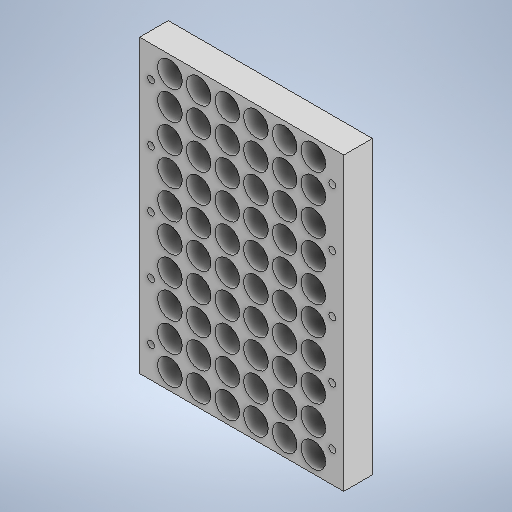
# Autodesk Inventor part: Battery Holder pt1
Saved by Autodesk Inventor 2025.2 (Build 292293000, 293)
## iProperties
Created: 2025-03-23
Part Number: Battery Holder pt1
Material: Generic
Document SubType Name: Modeling
Designer: Mathias
Density: 1 g/cm^3
Appearance: Default
Author: Mathias
Autodesk Inventor part; units mm, degrees
ref_plane "YZ Plane" through (0, 0, 0) normal (1, 0, 0) x (0, 1, 0)
ref_plane "XZ Plane" through (0, 0, 0) normal (0, 1, 0) x (-1, 0, 0)
ref_plane "XY Plane" through (0, 0, 0) normal (0, 0, 1) x (1, 0, 0)
sketch "Sketch1" plane through (0, 0, 0) normal (0, 0, 1) x (1, 0, 0)
  line L0 (0, 0) -> (178, 0)
  line L1 (178, 0) -> (178, 254)
  line L2 (178, 254) -> (0, 254)
  line L3 (0, 254) -> (0, 0)
  circle A0 centre (26.5, 14.5) radius 10.7
  circle A1 centre (26.5, 39.5) radius 10.7
  circle A2 centre (26.5, 64.5) radius 10.7
  circle A3 centre (26.5, 89.5) radius 10.7
  circle A4 centre (26.5, 114.5) radius 10.7
  circle A5 centre (26.5, 139.5) radius 10.7
  circle A6 centre (26.5, 164.5) radius 10.7
  circle A7 centre (26.5, 189.5) radius 10.7
  circle A8 centre (26.5, 214.5) radius 10.7
  circle A9 centre (26.5, 239.5) radius 10.7
  circle A10 centre (51.5, 14.5) radius 10.7
  circle A11 centre (51.5, 39.5) radius 10.7
  circle A12 centre (51.5, 64.5) radius 10.7
  circle A13 centre (51.5, 89.5) radius 10.7
  circle A14 centre (51.5, 114.5) radius 10.7
  circle A15 centre (51.5, 139.5) radius 10.7
  circle A16 centre (51.5, 164.5) radius 10.7
  circle A17 centre (51.5, 189.5) radius 10.7
  circle A18 centre (51.5, 214.5) radius 10.7
  circle A19 centre (51.5, 239.5) radius 10.7
  circle A20 centre (76.5, 14.5) radius 10.7
  circle A21 centre (76.5, 39.5) radius 10.7
  circle A22 centre (76.5, 64.5) radius 10.7
  circle A23 centre (76.5, 89.5) radius 10.7
  circle A24 centre (76.5, 114.5) radius 10.7
  circle A25 centre (76.5, 139.5) radius 10.7
  circle A26 centre (76.5, 164.5) radius 10.7
  circle A27 centre (76.5, 189.5) radius 10.7
  circle A28 centre (76.5, 214.5) radius 10.7
  circle A29 centre (76.5, 239.5) radius 10.7
  circle A30 centre (101.5, 14.5) radius 10.7
  circle A31 centre (101.5, 39.5) radius 10.7
  circle A32 centre (101.5, 64.5) radius 10.7
  circle A33 centre (101.5, 89.5) radius 10.7
  circle A34 centre (101.5, 114.5) radius 10.7
  circle A35 centre (101.5, 139.5) radius 10.7
  circle A36 centre (101.5, 164.5) radius 10.7
  circle A37 centre (101.5, 189.5) radius 10.7
  circle A38 centre (101.5, 214.5) radius 10.7
  circle A39 centre (101.5, 239.5) radius 10.7
  circle A40 centre (126.5, 14.5) radius 10.7
  circle A41 centre (126.5, 39.5) radius 10.7
  circle A42 centre (126.5, 64.5) radius 10.7
  circle A43 centre (126.5, 89.5) radius 10.7
  circle A44 centre (126.5, 114.5) radius 10.7
  circle A45 centre (126.5, 139.5) radius 10.7
  circle A46 centre (126.5, 164.5) radius 10.7
  circle A47 centre (126.5, 189.5) radius 10.7
  circle A48 centre (126.5, 214.5) radius 10.7
  circle A49 centre (126.5, 239.5) radius 10.7
  circle A50 centre (151.5, 14.5) radius 10.7
  circle A51 centre (151.5, 39.5) radius 10.7
  circle A52 centre (151.5, 64.5) radius 10.7
  circle A53 centre (151.5, 89.5) radius 10.7
  circle A54 centre (151.5, 114.5) radius 10.7
  circle A55 centre (151.5, 139.5) radius 10.7
  circle A56 centre (151.5, 164.5) radius 10.7
  circle A57 centre (151.5, 189.5) radius 10.7
  circle A58 centre (151.5, 214.5) radius 10.7
  circle A59 centre (151.5, 239.5) radius 10.7
  circle A60 centre (10, 27) radius 3
  circle A61 centre (10, 77) radius 3
  circle A62 centre (10, 127) radius 3
  circle A63 centre (10, 177) radius 3
  circle A64 centre (10, 227) radius 3
  circle A65 centre (168, 27) radius 3
  circle A66 centre (168, 77) radius 3
  circle A67 centre (168, 127) radius 3
  circle A68 centre (168, 177) radius 3
  circle A69 centre (168, 227) radius 3
  dimension "d0" = 178
  dimension "d1" = 254
  dimension "d2" = 21.4
  dimension "d5" = 25
  dimension "d8" = 25
  dimension "d31" = 6
  dimension "d34" = 50
  dimension "d37" = 158
  constraints: 70 centre point, 8 end point, 3 horizontal, 3 perpendicular, 2 vertical, 136 other
  measures "d0" distance of L0.start L0.end
  measures "d1" distance of L0.end L1.end
  measures "d2" diameter of A0
  measures "d5" distance of A0.centre A1.centre
  measures "d8" distance of A0.centre A10.centre
  measures "d31" diameter of A60
  measures "d34" distance of A60.centre A61.centre
  measures "d37" distance of A60.centre A65.centre
extrude "Extrusion1" add sketch "Sketch1" along normal blind 20
sketch "Sketch2" plane through (0, 0, 0) normal (0, 0, -1) x (-1, 0, 0)
  line L0 (-178, 0) -> (-178, 254) projected
  line L1 (-178, 254) -> (0, 254)
  line L2 (0, 254) -> (0, 0)
  line L3 (0, 0) -> (-178, 0)
  line L4 (-178, 0) -> (-178, 254)
  line L5 (-161, 5) -> (-92, 5)
  line L6 (-92, 5) -> (-92, 49)
  line L7 (-92, 49) -> (-161, 49)
  line L8 (-161, 49) -> (-161, 5)
  line L9 (-161, 99) -> (-161, 55)
  line L10 (-92, 99) -> (-161, 99)
  line L11 (-92, 55) -> (-92, 99)
  line L12 (-161, 55) -> (-92, 55)
  line L13 (-161, 149) -> (-161, 105)
  line L14 (-92, 149) -> (-161, 149)
  line L15 (-92, 105) -> (-92, 149)
  line L16 (-161, 105) -> (-92, 105)
  line L17 (-161, 199) -> (-161, 155)
  line L18 (-92, 199) -> (-161, 199)
  line L19 (-92, 155) -> (-92, 199)
  line L20 (-161, 155) -> (-92, 155)
  line L21 (-161, 249) -> (-161, 205)
  line L22 (-92, 249) -> (-161, 249)
  line L23 (-92, 205) -> (-92, 249)
  line L24 (-161, 205) -> (-92, 205)
  line L25 (-86, 49) -> (-86, 5)
  line L26 (-17, 49) -> (-86, 49)
  line L27 (-17, 5) -> (-17, 49)
  line L28 (-86, 5) -> (-17, 5)
  line L29 (-86, 99) -> (-86, 55)
  line L30 (-17, 99) -> (-86, 99)
  line L31 (-17, 55) -> (-17, 99)
  line L32 (-86, 55) -> (-17, 55)
  line L33 (-86, 149) -> (-86, 105)
  line L34 (-17, 149) -> (-86, 149)
  line L35 (-17, 105) -> (-17, 149)
  line L36 (-86, 105) -> (-17, 105)
  line L37 (-86, 199) -> (-86, 155)
  line L38 (-17, 199) -> (-86, 199)
  line L39 (-17, 155) -> (-17, 199)
  line L40 (-86, 155) -> (-17, 155)
  line L41 (-86, 249) -> (-86, 205)
  line L42 (-17, 249) -> (-86, 249)
  line L43 (-17, 205) -> (-17, 249)
  line L44 (-86, 205) -> (-17, 205)
  circle A0 centre (-168, 227) radius 3 projected
  circle A1 centre (-168, 227) radius 3
  circle A2 centre (-10, 227) radius 3
  circle A3 centre (-168, 177) radius 3
  circle A4 centre (-10, 177) radius 3
  circle A5 centre (-168, 127) radius 3
  circle A6 centre (-10, 127) radius 3
  circle A7 centre (-168, 77) radius 3
  circle A8 centre (-10, 77) radius 3
  circle A9 centre (-168, 27) radius 3
  circle A10 centre (-10, 27) radius 3
  dimension "d19" = 69
  dimension "d20" = 44
  dimension "d23" = 50
  dimension "d26" = 75
  dimension "d42" = 158
  dimension "d45" = 50
  constraints: 88 end point, 10 centre point, 4 horizontal, 4 parallel, 2 perpendicular, 2 vertical, 1 coincident, 90 other
  measures "d19" distance of L7.end L6.end
  measures "d20" distance of L6.end L5.end
  measures "d23" distance of L7.end L9.start
  measures "d26" distance of L7.end L25.start
  measures "d42" distance of A1.centre A2.centre
  measures "d45" distance of A1.centre A3.centre
extrude "Extrusion2" add sketch "Sketch2" along normal blind 5
body "Solid1"
